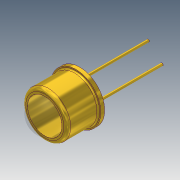
# Autodesk Inventor part: OD-110L
Saved by Autodesk Inventor 2015 SP1 (Build 190203100, 203)
## iProperties
Created: 2012-08-21
Material: ALUMINUM, 6061-T651
Vendor: DIGI-KEY
Document SubType Name: Modeling
Designer: COOPB
Mass: 0.99085 g
Surface Area: 3.53077 cm^2
Volume: 0.366981 cm^3
Density: 2.7 g/cm^3
Part Number: OD-110L
Project: P-25801
Description: IR EMITTER, 110mW, 850nm
Appearance: Gold Metallic
RuleStatus: InUse
AfterDocSave0: file://Part Number Cleaner
LAB/DEPT: COMMON
REQUESTING SCIENTIST: COMMON
SURFACE ROUGHNESS: N/A
DESIGN DEPARTMENT: HHMI: JFRC - ID&F
SPECIAL FINISH: NONE
ALTERED ITEM PART NUMBER: N/A
ALTERED ITEM VENDOR: N/A
ALTERED ITEM DESCRIPTION: N/A
Revision Number: A
Autodesk Inventor part; units mm, degrees
note: some values were not read from the file. Chosen so that the rebuilt part matches the saved one: pattern direction of "Circular Pattern1".
ref_plane "YZ Plane" through (0, 0, 0) normal (1, 0, 0) x (0, 1, 0)
ref_plane "XZ Plane" through (0, 0, 0) normal (0, 1, 0) x (-1, 0, 0)
ref_plane "XY Plane" through (0, 0, 0) normal (0, 0, 1) x (1, 0, 0)
sketch "Sketch1" plane through (0, 0, 0) normal (1, 0, 0) x (0, 1, 0)
  line L0 (0, 13.8497) -> (0, -17.125) projected
  line L1 (-0.9246, 0) -> (5.5474, 0) construction
  line L2 (4.6228, 0) -> (4.6228, 0.7112)
  line L3 (4.6228, 0.7112) -> (4.1656, 0.7112)
  line L4 (4.1656, 0.7112) -> (4.1656, 6.477)
  line L5 (4.1656, 6.477) -> (3.175, 6.477)
  arc A0 (3.175, 6.477) -> (0, 8.89) centre (0, 5.5947) ccw
  line L6 (4.6228, 0) -> (0, 0)
  line L7 (2.9972, 0) -> (2.54, 0)
  line L8 (2.54, 0) -> (2.54, -12.7)
  line L9 (2.54, -12.7) -> (2.7686, -12.7)
  line L10 (2.7686, -12.7) -> (2.7686, 0)
  line L11 (3.175, 6.477) -> (3.175, 1.016)
  line L12 (3.175, 1.016) -> (0, 1.016)
  point P0 (0, 6.477)
  dimension "d0" = 2.54
  dimension "d1" = 0.4572
  dimension "d2" = 12.7
  dimension "d3" = 0.7112
  dimension "d4" = 6.477
  dimension "d5" = 9.2456
  dimension "d6" = 8.3312
  dimension "d7" = 6.35
  dimension "d8" = 2.413
  dimension "d23" = 1.016
  constraints: 22 end point, 7 point on line, 5 perpendicular, 3 parallel, 2 point on circle, 1 centre point, 1 collinear, 1 midpoint
  measures "d0" distance between parallel lines of L0 L8
  measures "d1" diameter of L10 L8
  measures "d2" distance between parallel lines of L1 L9
  measures "d3" distance between parallel lines of L3 L1
  measures "d4" distance between parallel lines of L5 L1
  measures "d5" diameter of L2 L0
  measures "d6" diameter of L4 L0
  measures "d7" diameter of L5.end L0
  measures "d8" distance from line of A0.end L5
  measures "d23" distance between parallel lines of L6 L12
sketch "Sketch2" plane through (0, 0, 0) normal (0, 0, 1) x (1, 0, 0)
  line L0 (0, 6.4772) -> (0, -6.5034) construction
  line L1 (-6.5034, 0) -> (6.4772, 0) construction
  circle A0 centre (0, 0) radius 4.6228 construction
  line L2 (0, 0) -> (-4.6491, -4.6491) construction
  line L3 (-3.5271, -2.9883) -> (-4.1668, -3.628)
  line L4 (-4.1668, -3.628) -> (-3.628, -4.1668)
  line L5 (-3.628, -4.1668) -> (-2.9883, -3.5271)
  arc A1 (-3.5271, -2.9883) -> (-2.9883, -3.5271) centre (0, 0) ccw
  dimension "d9" = 9.2456
  dimension "d10" = 0.762
  dimension "d11" = 0.889
  dimension "d12" = 45
  constraints: 8 end point, 4 point on circle, 2 centre point, 2 coincident, 2 parallel, 1 perpendicular, 1 other
  measures "d9" diameter of A0
  measures "d10" distance between parallel lines of L3 L5
  measures "d11" distance edge to line of A0 L4
  measures "d12" angle of L1 L2
revolve "Revolution1" add sketch "Sketch1" angle 360 about axis through (0, 0, 0) along (0, 0, -1) contours L12 L11 L5 L4 L3 L2 L6 L0
revolve "Revolution2" add sketch "Sketch1" angle 360 about axis through (0, 2.54, 0) along (0, 0, -1) contours L6 L10 L9 L8
extrude "Extrusion1" add sketch "Sketch2" along normal up to surface (0.7112 mm away) from surface at 0
pattern_circular "Circular Pattern1" count 3 over 180 about axis through (0, 0, -10) along (0, 0, -1) of "Revolution2"
fillet "Fillet1" radius 0.635 1 edges at (0, -4.1656, 6.477)
fillet "Fillet1" radius 0.254 1 edges at (0, -4.1656, 0.7112)
revolve "Revolution3" add sketch "Sketch1" angle 360 about axis through (0, 0, 0) along (0, 0, -1) separate body contours A0 L11 L12 L0
equation "\"d9\" = d5"
body "Solid1"
body "Solid2"
